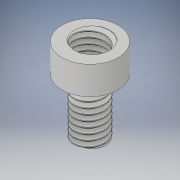
# Autodesk Inventor part: macho_y_hembra
Saved by Autodesk Inventor 2019 (Build 230136000, 136)
## iProperties
Created: 2018-12-22
Part Number: macho_y_hembra
Material: Generic
Document SubType Name: Modeling
Designer: assman
Density: 1 g/cm^3
Appearance: Default
Author: assman
Autodesk Inventor part; units mm, degrees
ref_plane "YZ Plane" through (0, 0, 0) normal (1, 0, 0) x (0, 1, 0)
ref_plane "XZ Plane" through (0, 0, 0) normal (0, 1, 0) x (-1, 0, 0)
ref_plane "XY Plane" through (0, 0, 0) normal (0, 0, 1) x (1, 0, 0)
sketch "Sketch1" plane through (0, 0, 0) normal (0, 1, 0) x (-1, 0, 0)
  circle A0 centre (0, 0) radius 5
  dimension "d0" = 10
  constraints: 1 centre point, 1 coincident
  measures "d0" diameter of A0
extrude "Extrusion1" add sketch "Sketch1" along normal blind 5
sketch "Sketch2" plane through (0, 5, 0) normal (0, 1, 0) x (1, 0, 0)
  circle A0 centre (0, 0) radius 5 projected
  constraints: 1 coincident
hole "Hole1" at (0, 5, 0) direction (0, -1, 0) diameter 7 end through all
thread "Thread1" size "M7x1" class "6H" standard "ANSI Metric M Profile" full length
sketch "Sketch4" plane through (0, 5, 0) normal (1, 0, 0) x (0, 0, 1)
  line L0 (3.5, 0) -> (3.5, 5)
  line L1 (3.5, 5) -> (2.7585, 5)
  line L2 (2.7585, 5) -> (2.7585, 0)
  line L3 (2.7585, 0) -> (3.5, 0)
  line L4 (0, -2.3086) -> (0, 6.2181) projected
  constraints: 8 end point
revolve "Revolution1" add sketch "Sketch4" angle 360 about axis through (0, 5, 0) along (0, -1, 0) separate body
sketch "Sketch3" plane through (0, 5, 3.5) normal (-1, 0, 0) x (0, -1, 0)
  line L0 (-0.5834, -0.0507) -> (-0.5001, -0.0507) construction
  line L1 (0.0832, -0.6911) -> (-0.0001, -0.8511) construction
  line L2 (-1.0001, -0.8511) -> (-1.0834, -0.6911) construction
  line L3 (-0.4168, -0.0507) -> (-0.5001, 0.1093) construction
  line L4 (-0.5001, 0.1093) -> (-0.5834, -0.0507) construction
  line L5 (-1.0001, -0.8511) -> (-0.9168, -0.6911) construction
  line L6 (-0.4168, -0.0507) -> (-0.0834, -0.6911)
  line L7 (-1.0834, -0.6911) -> (-0.9168, -0.6911) construction
  arc A0 (-1.0834, -0.6911) -> (-1.0001, -0.7416) centre (-1.0001, -0.6477) ccw construction
  line L8 (0.0832, -0.6911) -> (-0.0834, -0.6911) construction
  line L9 (-1.0001, -0.8511) -> (-1.0001, -0.6911) construction
  line L10 (-0.0001, -0.8511) -> (-0.0001, -0.6911) construction
  line L11 (-0.5001, 0.1093) -> (-0.5001, -0.0002) construction
  line L12 (-1.0001, -0.7416) -> (-0.0001, -0.7416)
  arc A1 (-1.0001, -0.7416) -> (-0.9168, -0.6911) centre (-1.0001, -0.6477) ccw
  line L13 (-0.0834, -0.6911) -> (-0.0001, -0.8511) construction
  line L14 (-0.9168, -0.6911) -> (-0.5834, -0.0507)
  line L15 (-0.0001, -0.0002) -> (-0.0001, 0.0177)
  line L16 (-0.0001, 0.0177) -> (-0.0001, -0.0002)
  line L17 (-0.0001, -0.0002) -> (0.0334, -0.0002)
  arc A2 (-0.0834, -0.6911) -> (-0.0001, -0.7416) centre (-0.0001, -0.6477) ccw
  arc A3 (-0.0001, -0.7416) -> (0.0832, -0.6911) centre (-0.0001, -0.6477) ccw construction
  arc A4 (-0.5001, -0.0002) -> (-0.5834, -0.0507) centre (-0.5001, -0.0941) ccw
  arc A5 (-0.4168, -0.0507) -> (-0.5001, -0.0002) centre (-0.5001, -0.0941) ccw
  line L18 (-0.5001, -0.0002) -> (-0.5001, -0.0507) construction
  line L19 (-0.5001, -0.0507) -> (-0.4168, -0.0507) construction
  dimension "d12" = 55
  dimension "d13" = 0.1601
  dimension "d14" = 0.1601
  dimension "Sketch3_ThreadOffset" = 0
  dimension "Sketch3_MajorRadius" = 0.7415
  dimension "d17" = 1
  dimension "Sketch3_MinorRadius" = 0
  constraints: 40 end point, 12 point on circle, 10 parallel, 8 tangent, 6 centre point, 6 collinear, 2 midpoint, 2 point on line, 1 horizontal, 1 perpendicular, 3 other
  measures "d12" angle of L6 L14
  measures "d13" distance of L3.end L0.end
  measures "d14" distance of L1.end L10.end
  measures "Sketch3_ThreadOffset" distance between parallel lines of L15 L10
  measures "Sketch3_MajorRadius" distance from line of L12 L15.start
  measures "d17" distance from line of L1.end L9
  measures "Sketch3_MinorRadius" distance edge to line of A5 L17
coil "Coil1" sketch "Sketch3" operation cut axis through (0, 5, 0) along (0, -1, 0) pitch 1.001 turns 6.993007 hand right bodies 2
combine bodies "Combine1" operation type add bodies to combine 2 1
sketch "Sketch6" plane through (0, 0, 0) normal (0, -1, 0) x (1, 0, 0)
  circle A0 centre (0, 0) radius 2.057
  dimension "d54" = 4.114
  constraints: 1 centre point, 1 coincident
  measures "d54" diameter of A0
sketch "Sketch9" plane through (0, -10, 0) normal (-1, 0, 0) x (0, 0, 1)
  line L0 (2.798, 0) -> (2.798, 10)
  line L1 (2.798, 10) -> (2.0565, 10)
  line L2 (2.0565, 10) -> (2.0565, 0)
  line L3 (2.0565, 0) -> (2.798, 0)
  line L4 (0, -4.3753) -> (0, 18.6181) projected
  constraints: 8 end point
revolve "Revolution2" cut sketch "Sketch9" angle 360 about axis through (0, -10, 0) along (0, 1, 0) bodies 1
sketch "Sketch10" plane through (0, -10, 0) normal (-1, 0, 0) x (0, 0, 1)
  line L0 (2.798, 0) -> (2.798, 10)
  line L1 (2.798, 10) -> (2.0565, 10)
  line L2 (2.0565, 10) -> (2.0565, 0)
  line L3 (2.0565, 0) -> (2.798, 0)
  line L4 (0, -4.3753) -> (0, 18.6181) projected
  constraints: 8 end point
revolve "Revolution3" add sketch "Sketch10" angle 360 about axis through (0, -10, 0) along (0, 1, 0) separate body
sketch "Sketch8" plane through (0, -10, 0) normal (1, 0, 0) x (0, 1, 0)
  line L0 (-0.5834, -2.1073) -> (-0.5001, -2.1073) construction
  line L1 (0.0832, -2.7476) -> (-0.0001, -2.9077) construction
  line L2 (-1.0001, -2.9077) -> (-1.0834, -2.7476) construction
  line L3 (-0.4168, -2.1073) -> (-0.5001, -1.9472) construction
  line L4 (-0.5001, -1.9472) -> (-0.5834, -2.1073) construction
  line L5 (-1.0001, -2.9077) -> (-0.9168, -2.7476) construction
  line L6 (-0.4168, -2.1073) -> (-0.0834, -2.7476)
  line L7 (-1.0834, -2.7476) -> (-0.9168, -2.7476) construction
  arc A0 (-1.0834, -2.7476) -> (-1.0001, -2.7982) centre (-1.0001, -2.7042) ccw construction
  line L8 (0.0832, -2.7476) -> (-0.0834, -2.7476) construction
  line L9 (-1.0001, -2.9077) -> (-1.0001, -2.7476) construction
  line L10 (-0.0001, -2.9077) -> (-0.0001, -2.7476) construction
  line L11 (-0.5001, -1.9472) -> (-0.5001, -2.0567) construction
  line L12 (-1.0001, -2.7982) -> (-0.0001, -2.7982)
  arc A1 (-1.0001, -2.7982) -> (-0.9168, -2.7476) centre (-1.0001, -2.7042) ccw
  line L13 (-0.0834, -2.7476) -> (-0.0001, -2.9077) construction
  line L14 (-0.9168, -2.7476) -> (-0.5834, -2.1073)
  line L15 (-0.0001, -0.0002) -> (-0.0001, 0.0177)
  line L16 (-0.0001, 0.0177) -> (-0.0001, -0.0002)
  line L17 (-0.0001, -0.0002) -> (0.0334, -0.0002)
  arc A2 (-0.0834, -2.7476) -> (-0.0001, -2.7982) centre (-0.0001, -2.7042) ccw
  arc A3 (-0.0001, -2.7982) -> (0.0832, -2.7476) centre (-0.0001, -2.7042) ccw construction
  arc A4 (-0.5001, -2.0567) -> (-0.5834, -2.1073) centre (-0.5001, -2.1507) ccw
  arc A5 (-0.4168, -2.1073) -> (-0.5001, -2.0567) centre (-0.5001, -2.1507) ccw
  line L18 (-0.5001, -2.0567) -> (-0.5001, -2.1073) construction
  line L19 (-0.5001, -2.1073) -> (-0.4168, -2.1073) construction
  dimension "d35" = 55
  dimension "d36" = 0.1601
  dimension "d37" = 0.1601
  dimension "Sketch8_ThreadOffset" = 0
  dimension "Sketch8_MajorRadius" = 2.798
  dimension "d40" = 1
  dimension "Sketch8_MinorRadius" = 2.0565
  constraints: 40 end point, 12 point on circle, 10 parallel, 8 tangent, 6 centre point, 6 collinear, 2 midpoint, 2 point on line, 1 horizontal, 1 perpendicular, 3 other
  measures "d35" angle of L6 L14
  measures "d36" distance of L3.end L0.end
  measures "d37" distance of L1.end L10.end
  measures "Sketch8_ThreadOffset" distance between parallel lines of L15 L10
  measures "Sketch8_MajorRadius" distance from line of L12 L15.start
  measures "d40" distance from line of L1.end L9
  measures "Sketch8_MinorRadius" distance edge to line of A5 L17
coil "Coil2" sketch "Sketch8" operation cut axis through (0, -10, 0) along (0, 1, 0) pitch 1.001 turns 11.988012 hand right bodies 3
extrude "Extrusion3" add sketch "Sketch6" along normal blind 10 separate body
combine bodies "Combine2" operation type add bodies to combine 3 4
equation "\"d12\" = d19"
equation "\"d13\" = 0.160083 * Sketch3_Pitch"
equation "\"d14\" = 0.160083 * Sketch3_Pitch"
equation "\"d17\" = Sketch3_Pitch"
equation "\"d35\" = d42"
equation "\"d36\" = 0.160083 * Sketch8_Pitch"
equation "\"d37\" = 0.160083 * Sketch8_Pitch"
equation "\"d40\" = Sketch8_Pitch"
equation "\"d19\" = 55deg"
equation "\"Sketch3_Pitch\" = 1"
equation "\"d42\" = 55deg"
equation "\"Sketch8_Pitch\" = 1"
body "Solid1"
body "Solid5"
